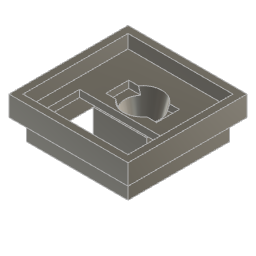
Jet Select Buttons v2 (Autodesk Fusion 360 design; units mm, degrees)
Autodesk Fusion 360 part; units mm, degrees
sketch "Sketch1" plane through (0, 0, 0) normal (0, 1, 0) x (1, 0, 0) in component "PUSH BUTTON SUPPORT v7"
  line L0 (2.815, 2.25) -> (-2.815, 2.25)
  line L1 (-2.815, 2.25) -> (-2.815, -2.25)
  line L2 (-2.815, -2.25) -> (2.815, -2.25)
  line L3 (2.815, -2.25) -> (2.815, 2.25)
  line L4 (2.815, 2.25) -> (-2.815, -2.25) construction
  line L5 (-2.815, 2.25) -> (2.815, -2.25) construction
  line L6 (3.815, 3.25) -> (-3.815, 3.25)
  line L7 (-3.815, 3.25) -> (-3.815, -3.25)
  line L8 (-3.815, -3.25) -> (3.815, -3.25)
  line L9 (3.815, -3.25) -> (3.815, 3.25)
  line L10 (3.815, 3.25) -> (-3.815, -3.25) construction
  line L11 (-3.815, 3.25) -> (3.815, -3.25) construction
  line L12 (1, 1.85) -> (-1, 1.85)
  line L13 (1, 1.85) -> (-1, -1.85) construction
  line L14 (-1, 1.85) -> (1, -1.85) construction
  line L15 (-0.994265, -2.25) -> (1, -2.25)
  line L16 (1, -2.25) -> (1, -1.85)
  line L17 (1, -1.85) -> (-0.994265, -1.85)
  line L18 (-0.994265, -1.85) -> (-0.994265, -2.25)
  line L19 (1, 1.85) -> (1, 2.25)
  line L20 (1, 2.25) -> (-1, 2.25)
  line L21 (-1, 2.25) -> (-1, 1.85)
  line L22 (-2.815, -2.25) -> (-2.515, -2.25)
  line L23 (-2.515, -2.25) -> (-2.515, 2.25)
  line L24 (-2.515, 2.25) -> (-2.815, 2.25)
  line L25 (-2.815, 2.25) -> (-2.815, -2.25)
  line L26 (2.815, -2.25) -> (2.515, -2.25)
  line L27 (2.515, -2.25) -> (2.515, 2.25)
  line L28 (2.515, 2.25) -> (2.815, 2.25)
  line L29 (2.815, 2.25) -> (2.815, -2.25)
  dimension "d1" = 5.63
  dimension "d2" = 4.5
  dimension "d3" = 7.63
  dimension "d4" = 6.5
  dimension "d7" = 2
  dimension "d8" = 3.7
  dimension "d11" = 0.3
  dimension "d12" = 0.3
  constraint horizontal L0
  constraint perpendicular L0 L1
  constraint parallel L0 L2
  constraint parallel L1 L3
  constraint coincident L4 origin
  constraint coincident L5 origin
  constraint horizontal L6
  constraint perpendicular L6 L7
  constraint parallel L6 L8
  constraint parallel L7 L9
  constraint coincident L10 origin
  constraint coincident L11 origin
  constraint horizontal L12
  constraint coincident L13 origin
  constraint coincident L14 origin
  constraint horizontal L15
  constraint vertical L16
  constraint horizontal L17
  constraint vertical L18
  constraint vertical L19
  constraint horizontal L20
  constraint vertical L21
  constraint coincident L0 L19.end
  constraint horizontal L22
  constraint vertical L23
  constraint horizontal L24
  constraint vertical L25
  constraint horizontal L26
  constraint vertical L27
  constraint horizontal L28
  constraint vertical L29
  measures "d1" distance of L1.end L2.end
  measures "d2" distance of L0.end L1.end
  measures "d3" distance of L7.end L8.end
  measures "d4" distance of L6.end L7.end
  measures "d7" distance of L13.end L14.end
  measures "d8" distance of L12.end L13.end
  measures "d11" distance of L1.end L22.end
  measures "d12" distance of L2.end L26.end
extrude "Extrude1" add sketch "Sketch1" along normal blind 5 contours L6 L7 L8 L9 picked at (-0.331422, -2.916667) in component "PUSH BUTTON SUPPORT v7"
extrude "Extrude2" add sketch "Sketch1" along normal blind 5 contours L0 L12 L19 L20 L21 | L2 L15 L16 L17 L18 picked at (-0.333333, 2.116667) picked at (0.335245, -2.116667) in component "PUSH BUTTON SUPPORT v7"
extrude "Extrude3" add sketch "Sketch1" along normal blind 1.8 contours L0 L2 L3 L26 L27 L28 L29 | L0 L1 L2 L22 L23 L24 L25 picked at (2.615, 0.75) picked at (-2.715, 0.75) in component "PUSH BUTTON SUPPORT v7"
chamfer "Chamfer1" distance 0.3 angle 45 2 edges at (-2.515, 1.8, 0) (2.515, 1.8, 0) in component "PUSH BUTTON SUPPORT v7"
chamfer "Chamfer3" distance 0.9 distance2 0.3 1 edges at (-2.515, 0, 0) measured on face at (-2.515, 0.50002, 0.75) in component "PUSH BUTTON SUPPORT v7"
chamfer "Chamfer4" distance 0.3 distance2 1 1 edges at (2.515, 0, 0) measured on face at (3.381667, 0, 0.75) in component "PUSH BUTTON SUPPORT v7"
sketch "Sketch2" plane through (0, 0, 3.25) normal (0, 0, 1) x (-1, 0, 0) in component "PUSH BUTTON SUPPORT v7"
  line L0 (3.815, 0) -> (-3.815, 0)
  line L1 (-3.815, 0) -> (-3.815, -5)
  line L2 (-3.815, -5) -> (3.815, -5)
  line L3 (3.815, -5) -> (3.815, 0)
  line L4 (-2.81825, -1.967525) -> (2.836671, -1.967525)
  line L5 (2.836671, -1.967525) -> (2.836671, -2.718821)
  line L6 (2.836671, -2.718821) -> (-2.81825, -2.718821)
  line L7 (-2.81825, -2.718821) -> (-2.81825, -1.967525)
  constraint horizontal L4
  constraint vertical L5
  constraint horizontal L6
  constraint vertical L7
extrude "Extrude4" add sketch "Sketch2" against normal blind 6.5 contours L4 L5 L6 L7 picked at (-0.933276, -2.217957) in component "PUSH BUTTON SUPPORT v7"
sketch "Sketch3" plane through (0, 1.967525, 0) normal (0, -1, 0) x (1, 0, 0) in component "PUSH BUTTON SUPPORT v7"
  line L0 (-1, -1.85) -> (1, -1.85)
  line L1 (1, -1.85) -> (1, -2.25)
  line L2 (1, -2.25) -> (2.815, -2.25)
  line L3 (2.815, -2.25) -> (2.815, 2.25)
  line L4 (2.815, 2.25) -> (1, 2.25)
  line L5 (1, 2.25) -> (1, 1.85)
  line L6 (1, 1.85) -> (-0.994265, 1.85)
  line L7 (-0.994265, 1.85) -> (-0.994265, 2.25)
  line L8 (-0.994265, 2.25) -> (-2.815, 2.25)
  line L9 (-2.815, 2.25) -> (-2.815, -2.25)
  line L10 (-2.815, -2.25) -> (-1, -2.25)
  line L11 (-1, -2.25) -> (-1, -1.85)
  circle A0 centre (0, 0) radius 1.019835
  constraint coincident A0.centre origin
extrude "Extrude5" cut sketch "Sketch3" against normal blind 6.5 contours A0 picked at (-0.371624, 0.422719) in component "PUSH BUTTON SUPPORT v7"
extrude "Extrude6" cut 1 faces at (-0.331422, 5, 2.916667) along direction (0, -1, 0) blind 2 in component "PUSH BUTTON SUPPORT v7"
extrude "Extrude7" cut 1 faces at (1, 0.655842, -1.983333) along direction (-1, 0, 0) blind 0.3 in component "PUSH BUTTON SUPPORT v7"
extrude "Extrude8" cut 1 faces at (1, 0.655842, 2.116667) along direction (-1, 0, 0) blind 0.3 in component "PUSH BUTTON SUPPORT v7"
extrude "Extrude9" cut 1 faces at (-1, 0.655842, -2.116667) along direction (1, 0, 0) blind 0.3 in component "PUSH BUTTON SUPPORT v7"
extrude "Extrude10" cut 1 faces at (-0.994265, 0.655842, 1.983333) along direction (1, 0, 0) blind 0.3 in component "PUSH BUTTON SUPPORT v7"
extrude "Extrude11" cut 2 faces at (-1.305, 0.955842, -2.25) (1.305, 0.989175, -2.25) along direction (0, 0, -1) blind 0.3 in component "PUSH BUTTON SUPPORT v7"
extrude "Extrude12" cut 2 faces at (-1.301176, 0.955842, 2.25) (1.305, 0.989175, 2.25) along direction (0, 0, 1) blind 0.3 in component "PUSH BUTTON SUPPORT v7"
extrude "Extrude13" cut 1 faces at (-3.481667, 0, -0.85) along direction (0, 1, 0) blind 0.5 in component "PUSH BUTTON SUPPORT v7"
extrude "Extrude14" cut 1 faces at (-2.815, 0.166667, -0.85) along direction (1, 0, 0) blind 8 in component "PUSH BUTTON SUPPORT v7"
extrude "Extrude15" cut 2 faces at (2.81498, 1.8, 0.85) (2.71496, 1.70002, -0.85) along direction (0.70710678, -0.70710678, 0) blind 0.3 in component "PUSH BUTTON SUPPORT v7"
extrude "Extrude16" cut 2 faces at (-2.81498, 1.8, -0.85) (-2.71496, 1.70002, -0.85) along direction (-0.70710678, -0.70710678, 0) blind 0.3 in component "PUSH BUTTON SUPPORT v7"
extrude "Extrude17" cut 1 faces at (2.565, 0.833333, 0.85) along direction (0.95782629, 0.28734789, 0) blind 0.1 in component "PUSH BUTTON SUPPORT v7"
extrude "Extrude18" cut 1 faces at (-2.559444, 0.766667, 0.85) along direction (-0.9486833, 0.31622777, 0) blind 0.1 in component "PUSH BUTTON SUPPORT v7"
extrude "Extrude19" cut 1 faces at (2.515, 1.166687, 0.85) along direction (1, 0, 0) blind 0.1 in component "PUSH BUTTON SUPPORT v7"
extrude "Extrude20" cut 1 faces at (-2.515, 1.10002, 0.85) along direction (-1, 0, 0) blind 0.1 in component "PUSH BUTTON SUPPORT v7"
extrude "Extrude21" cut 1 faces at (-2.815, 1.911683, -0.85) along direction (-1, 0, 0) blind 0.2 in component "PUSH BUTTON SUPPORT v7"
extrude "Extrude22" cut 1 faces at (2.815, 1.911683, -0.85) along direction (1, 0, 0) blind 0.2 in component "PUSH BUTTON SUPPORT v7"
extrude "Extrude23" cut 1 faces at (-0.7, 0.989175, -2.316667) along direction (1, 0, 0) blind 0.5 in component "PUSH BUTTON SUPPORT v7"
extrude "Extrude24" cut 1 faces at (-0.694265, 1.47835, 2.316667) along direction (1, 0, 0) blind 0.5 in component "PUSH BUTTON SUPPORT v7"
extrude "Extrude25" cut 1 faces at (0.7, 0.989175, 2.316667) along direction (-1, 0, 0) blind 0.5 in component "PUSH BUTTON SUPPORT v7"
extrude "Extrude26" cut 1 faces at (0.7, 1.47835, -2.316667) along direction (-1, 0, 0) blind 0.5 in component "PUSH BUTTON SUPPORT v7"
extrude "Extrude27" cut 1 faces at (0.068578, 0.989175, 1.85) along direction (0, 0, 1) blind 0.2 in component "PUSH BUTTON SUPPORT v7"
extrude "Extrude28" cut 1 faces at (0.066667, 0.989175, -1.85) along direction (0, 0, -1) blind 0.2 in component "PUSH BUTTON SUPPORT v7"
extrude "Extrude29" cut 2 faces at (1.005, 1.289195, -2.55) (-1.005, 1.289195, -2.55) along direction (0, 0, -1) blind 0.1 in component "PUSH BUTTON SUPPORT v7"
extrude "Extrude30" cut 2 faces at (-1.001176, 1.289195, 2.55) (1.005, 1.289195, 2.55) along direction (0, 0, 1) blind 0.1 in component "PUSH BUTTON SUPPORT v7"
chamfer "Chamfer2" [suppressed] in component "PUSH BUTTON SUPPORT v7"
sketch "Sketch1 (2)" plane through (0, 0, 0.878877) normal (0, 0, 1) x (-1, 0, 0)
  circle A0 centre (0, -1.839996) radius 1.019835
  line L0 (-1, -3.689996) -> (1, -3.689996)
  line L1 (1, -3.689996) -> (1, -4.089996)
  line L2 (1, -4.089996) -> (2.815, -4.089996)
  line L3 (2.815, -4.089996) -> (2.815, 0.410004)
  line L4 (2.815, 0.410004) -> (0.994265, 0.410004)
  line L5 (0.994265, 0.410004) -> (0.994265, 0.010004)
  line L6 (0.994265, 0.010004) -> (-1, 0.010004)
  line L7 (-1, 0.010004) -> (-1, 0.410004)
  line L8 (-1, 0.410004) -> (-2.815, 0.410004)
  line L9 (-2.815, 0.410004) -> (-2.815, -4.089996)
  line L10 (-2.815, -4.089996) -> (-1, -4.089996)
  line L11 (-1, -4.089996) -> (-1, -3.689996)
  line L12 (2.815, -4.089996) -> (-2.815, -4.089996)
  line L13 (-2.815, -4.089996) -> (-2.815, 0.410004)
  line L14 (-2.815, 0.410004) -> (2.815, 0.410004)
  line L15 (2.815, 0.410004) -> (2.815, -4.089996)
  circle A1 centre (0, -1.839996) radius 1.019835
  constraint horizontal L12
  constraint vertical L13
  constraint horizontal L14
  constraint vertical L15
extrude "Extrude31" add sketch "Sketch1 (2)" along normal blind 0.281 contours L0 L1 L2 L3 L4 L5 L6 L7 L8 L9 L10 L11 L12 L13 L14 L15 picked at (-2.216612, -1.839996) sketch seen with x (1, 0, 0) y (0, 0, -1) z (0, 1, 0) at (0, 1.839944, 1.839996) in component "PUSH BUTTON SUPPORT v7"
sketch "Sketch2 (2)" plane through (0, 0, 1.160056) normal (0, 0, 1) x (-1, 0, 0)
  line L0 (-2.815, -4.089996) -> (-2.815, 0.410004)
  line L1 (-2.815, 0.410004) -> (-1, 0.410004)
  line L2 (-1, 0.410004) -> (-1, 0.010004)
  line L3 (-1, 0.010004) -> (0.994265, 0.010004)
  line L4 (0.994265, 0.010004) -> (0.994265, 0.410004)
  line L5 (0.994265, 0.410004) -> (2.815, 0.410004)
  line L6 (2.815, 0.410004) -> (2.815, -4.089996)
  line L7 (2.815, -4.089996) -> (1, -4.089996)
  line L8 (1, -4.089996) -> (1, -3.689996)
  line L9 (1, -3.689996) -> (-1, -3.689996)
  line L10 (-1, -3.689996) -> (-1, -4.089996)
  line L11 (-1, -4.089996) -> (-2.815, -4.089996)
  line L12 (-3.815, 1.410004) -> (-3.815, -5.089996)
  line L13 (-3.815, -5.089996) -> (3.815, -5.089996)
  line L14 (3.815, -5.089996) -> (3.815, 1.410004)
  line L15 (3.815, 1.410004) -> (-3.815, 1.410004)
  line L16 (0.003684, -1.88932) -> (2.866211, -1.88932)
  line L17 (2.866211, -1.88932) -> (2.866211, -7.811173)
  line L18 (2.866211, -7.811173) -> (0.003684, -7.811173)
  line L19 (0.003684, -7.811173) -> (0.003684, -1.88932)
  line L20 (0.003684, -1.88932) -> (-1.123776, -1.88932)
  line L21 (-1.123776, -1.88932) -> (-1.123776, 8.11068)
  line L22 (-1.123776, 8.11068) -> (0.003684, 8.11068)
  line L23 (0.003684, 8.11068) -> (0.003684, -1.88932)
  line L24 (-4.246316, 1.795447) -> (4.253684, 1.795447)
  line L25 (4.253684, 1.795447) -> (4.253684, -5.574087)
  line L26 (4.253684, -5.574087) -> (-4.246316, -5.574087)
  line L27 (-4.246316, -5.574087) -> (-4.246316, 1.795447)
  line L28 (-4.246316, 1.795447) -> (4.253684, -5.574087) construction
  line L29 (4.253684, 1.795447) -> (-4.246316, -5.574087) construction
  line L30 (8.540865, -7.770507) -> (-8.459135, -7.770507)
  line L31 (-8.459135, -7.770507) -> (-8.459135, 9.229493)
  line L32 (-8.459135, 9.229493) -> (8.540865, 9.229493)
  line L33 (8.540865, 9.229493) -> (8.540865, -7.770507)
  point P0 (0.003684, -1.88932)
  dimension "d78" = 10
  dimension "d79" = 8.5
  dimension "d80" = 17
  dimension "d81" = 17
  constraint horizontal L16
  constraint vertical L17
  constraint horizontal L18
  constraint vertical L19
  constraint horizontal L20
  constraint vertical L21
  constraint horizontal L22
  constraint vertical L23
  constraint horizontal L24
  constraint perpendicular L24 L25
  constraint parallel L24 L26
  constraint parallel L25 L27
  constraint horizontal L30
  constraint vertical L31
  constraint horizontal L32
  constraint vertical L33
extrude "Extrude32" add sketch "Sketch2 (2)" along normal blind 4 contours L0 L1 L9 L10 L11 L12 L13 L15 L19 L21 | L0 L1 L9 L10 L11 L19 L20 L21 | L1 L2 L3 L15 L21 L23 | L1 L2 L3 L20 L21 L23 | L15 L21 L23 L24 | L12 L13 L15 L19 L21 L24 L26 L27 | L6 L7 L8 L9 L16 L19 | L6 L7 L8 L9 L13 L16 L17 L19 | L3 L4 L5 L6 L16 L23 | L13 L14 L15 L17 L23 L24 L25 L26 | L3 L4 L5 L6 L13 L14 L15 L16 L17 L23 | L17 L19 L21 L22 L23 L24 L25 L26 L27 L30 L31 L32 L33 | L21 L22 L23 L24 | L13 L17 L19 L26 | L17 L19 L26 L30 picked at (-3.481667, -1.089996) picked at (-2.251259, -1.856437) picked at (-0.330878, 0.610004) picked at (-0.706697, -1.256212) picked at (-0.372136, 1.538485) picked at (-2.685878, -5.412723) picked at (1.272895, -2.489545) picked at (1.289965, -4.756662) picked at (1.270983, -1.256212) picked at (4.107456, -2.956212) picked at (3.498737, -1.856437) picked at (4.266077, 6.37854) picked at (-0.372136, 6.005602) picked at (0.957859, -5.251359) picked at (1.912035, -7.038367) sketch seen with x (1, 0, 0) y (0, 0, -1) z (0, 1, 0) at (0, 1.839944, 1.839996) in component "PUSH BUTTON SUPPORT v7"
extrude "Extrude33" cut 1 faces at (-1.29891, 3, 8.462992) along direction (0, 1, 0) blind 3 in component "PUSH BUTTON SUPPORT v7"
extrude "Extrude34" cut 1 faces at (2.792469, 6.333333, 11.069488) along direction (0, 0, -1) blind 0.5 in component "PUSH BUTTON SUPPORT v7"
extrude "Extrude35" add 1 faces at (-2.874198, 6.333333, -5.930512) along direction (0, 0, -1) blind 0.5 in component "PUSH BUTTON SUPPORT v7"
sketch "Sketch3 (2)" plane through (0, 0, 5.160056) normal (0, 0, 1) x (-1, 0, 0)
  line L0 (8.540865, 8.729493) -> (-8.459135, 8.729493)
  line L1 (-8.459135, 8.729493) -> (-8.459135, -8.270507)
  line L2 (-8.459135, -8.270507) -> (8.540865, -8.270507)
  line L3 (8.540865, -8.270507) -> (8.540865, 8.729493)
  line L4 (5.982549, 1.207457) -> (-6.017451, 1.207457)
  line L5 (-6.017451, 1.207457) -> (-6.017451, 7.707457)
  line L6 (-6.017451, 7.707457) -> (5.982549, 7.707457)
  line L7 (5.982549, 7.707457) -> (5.982549, 1.207457)
  line L8 (5.982549, 1.207457) -> (-6.017451, 7.707457) construction
  line L9 (-6.017451, 1.207457) -> (5.982549, 7.707457) construction
  point P0 (-0.017451, 4.457457)
  dimension "d90" = 12
  dimension "d91" = 6.5
  constraint horizontal L4
  constraint perpendicular L4 L5
  constraint parallel L4 L6
  constraint parallel L5 L7
extrude "Extrude36" cut sketch "Sketch3 (2)" against normal blind 1 contours L4 L5 L6 L7 picked at (1.982549, 3.374123) sketch seen with x (1, 0, 0) y (0, 0, -1) z (0, 1, 0) at (0, 1.839944, 1.839996) in component "PUSH BUTTON SUPPORT v7"
sketch "Sketch4" plane through (0, 0, 5.160056) normal (0, 0, 1) x (-1, 0, 0)
  line L0 (-6.017451, 1.207457) -> (-6.017451, 7.707457)
  line L1 (-6.017451, 7.707457) -> (5.982549, 7.707457)
  line L2 (5.982549, 7.707457) -> (5.982549, 1.207457)
  line L3 (5.982549, 1.207457) -> (-6.017451, 1.207457)
  line L4 (8.540865, 8.729493) -> (-8.459135, 8.729493)
  line L5 (-8.459135, 8.729493) -> (-8.459135, -8.270507)
  line L6 (-8.459135, -8.270507) -> (8.540865, -8.270507)
  line L7 (8.540865, -8.270507) -> (8.540865, 8.729493)
  circle A0 centre (-0.005434, -1.819158) radius 1.75
  dimension "d94" = 3.5
  measures "d94" diameter of A0
extrude "Extrude37" cut sketch "Sketch4" against normal blind 6 contours A0 picked at (-0.585359, -1.346886) sketch seen with x (1, 0, 0) y (0, 0, -1) z (0, 1, 0) at (0, 1.839944, 1.839996) in component "PUSH BUTTON SUPPORT v7"
sketch "Sketch5" plane through (0, 0, 5.160056) normal (0, 0, 1) x (-1, 0, 0)
  circle A0 centre (-0.005434, -1.819158) radius 1.75
  line L0 (-6.017451, 1.207457) -> (-6.017451, 7.707457)
  line L1 (-6.017451, 7.707457) -> (5.982549, 7.707457)
  line L2 (5.982549, 7.707457) -> (5.982549, 1.207457)
  line L3 (5.982549, 1.207457) -> (-6.017451, 1.207457)
  line L4 (8.540865, 8.729493) -> (-8.459135, 8.729493)
  line L5 (-8.459135, 8.729493) -> (-8.459135, -8.270507)
  line L6 (-8.459135, -8.270507) -> (8.540865, -8.270507)
  line L7 (8.540865, -8.270507) -> (8.540865, 8.729493)
  line L8 (8.540865, -8.270507) -> (-8.459135, -8.270507)
  line L9 (-8.459135, -8.270507) -> (-8.459135, 8.729493)
  line L10 (-8.459135, 8.729493) -> (8.540865, 8.729493)
  line L11 (8.540865, 8.729493) -> (8.540865, -8.270507)
  line L12 (8.540865, -8.270507) -> (-8.459135, 8.729493)
  line L13 (-8.459135, -8.270507) -> (8.540865, 8.729493)
  line L14 (7.540865, -7.270507) -> (-7.459135, -7.270507)
  line L15 (-7.459135, -7.270507) -> (-7.459135, 7.729493)
  line L16 (-7.459135, 7.729493) -> (7.540865, 7.729493)
  line L17 (7.540865, 7.729493) -> (7.540865, -7.270507)
  line L18 (7.540865, -7.270507) -> (-7.459135, 7.729493) construction
  line L19 (-7.459135, -7.270507) -> (7.540865, 7.729493) construction
  point P0 (0.040865, 0.229493)
  dimension "d97" = 15
  dimension "d98" = 15
  constraint horizontal L8
  constraint vertical L9
  constraint horizontal L10
  constraint vertical L11
  constraint horizontal L14
  constraint perpendicular L14 L15
  constraint parallel L14 L16
  constraint parallel L15 L17
extrude "Extrude38" add sketch "Sketch5" along normal blind 1.9 contours L7 L11 L12 L13 L17 | L6 L8 L12 L13 L14 | L5 L9 L12 L13 L15 | L4 L10 L12 L13 L16 picked at (8.207531, -2.270507) picked at (-2.459135, -7.937174) picked at (-8.125802, 2.729493) picked at (-2.459135, 8.396159) sketch seen with x (1, 0, 0) y (0, 0, -1) z (0, 1, 0) at (0, 1.839944, 1.839996) in component "PUSH BUTTON SUPPORT v7"
extrude "Extrude39" add 1 faces at (2.017451, 6.666667, 9.547452) along direction (0, 0, -1) blind 1 in component "PUSH BUTTON SUPPORT v7"
chamfer "Chamfer5" distance 1 distance2 4 1 edges at (1.637007, 7, 0.653665) measured on face at (-5.082811, 7, -0.874348) in component "PUSH BUTTON SUPPORT v7"
sketch "Sketch6" plane through (0, 0, 5.160056) normal (0, 0, 1) x (-1, 0, 0)
  line L0 (-6.017451, 1.207457) -> (-6.017451, 6.707457)
  line L1 (-6.017451, 6.707457) -> (5.982549, 6.707457)
  line L2 (5.982549, 6.707457) -> (5.982549, 1.207457)
  line L3 (5.982549, 1.207457) -> (-6.017451, 1.207457)
  line L4 (-7.459135, 7.729493) -> (-7.459135, -7.270507)
  line L5 (-7.459135, -7.270507) -> (7.540865, -7.270507)
  line L6 (7.540865, -7.270507) -> (7.540865, 7.729493)
  line L7 (7.540865, 7.729493) -> (-7.459135, 7.729493)
  circle A0 centre (-0.005434, -1.819158) radius 2.75
  line L8 (3.614753, -3.441837) -> (-3.625622, -3.441837)
  line L9 (-3.625622, -3.441837) -> (-3.625622, -0.196479)
  line L10 (-3.625622, -0.196479) -> (3.614753, -0.196479)
  line L11 (3.614753, -0.196479) -> (3.614753, -3.441837)
  line L12 (3.614753, -3.441837) -> (-3.625622, -0.196479) construction
  line L13 (-3.625622, -3.441837) -> (3.614753, -0.196479) construction
  point P0 (-0.005434, -1.819158)
  constraint horizontal L8
  constraint perpendicular L8 L9
  constraint parallel L8 L10
  constraint parallel L9 L11
extrude "Extrude40" cut sketch "Sketch6" against normal blind 1 contours A0 L8 L10 | A0 L8 L10 L11 | A0 L8 L9 L10 picked at (-0.80412, -1.149714) picked at (3.32469, -1.819158) picked at (-3.333306, -1.754928) sketch seen with x (1, 0, 0) y (0, 0, -1) z (0, 1, 0) at (0, 1.839944, 1.839996) in component "PUSH BUTTON SUPPORT v7"
sketch "Sketch7" plane through (0, 0, 4.160056) normal (0, 0, -1) x (1, 0, 0)
  line L0 (6.017451, 1.207457) -> (3.815, 1.207457)
  line L1 (3.815, 1.207457) -> (3.815, -5.089996)
  line L2 (3.815, -5.089996) -> (-3.815, -5.089996)
  line L3 (-3.815, -5.089996) -> (-3.815, 1.207457)
  line L4 (-3.815, 1.207457) -> (-5.982549, 1.207457)
  line L5 (-5.982549, 1.207457) -> (-5.982549, 6.707457)
  line L6 (-5.982549, 6.707457) -> (6.017451, 6.707457)
  line L7 (6.017451, 6.707457) -> (6.017451, 1.207457)
  line L8 (8.459135, 8.729493) -> (-8.540865, 8.729493)
  line L9 (-8.540865, 8.729493) -> (-8.540865, -8.270507)
  line L10 (-8.540865, -8.270507) -> (8.459135, -8.270507)
  line L11 (8.459135, -8.270507) -> (8.459135, 8.729493)
  line L12 (-8.540865, 8.729493) -> (8.459135, -8.270507)
  line L13 (8.459135, 8.729493) -> (-8.540865, -8.270507)
  line L14 (-7.290865, 7.479493) -> (7.209135, 7.479493)
  line L15 (7.209135, 7.479493) -> (7.209135, -7.020507)
  line L16 (7.209135, -7.020507) -> (-7.290865, -7.020507)
  line L17 (-7.290865, -7.020507) -> (-7.290865, 7.479493)
  line L18 (-7.290865, 7.479493) -> (7.209135, -7.020507) construction
  line L19 (7.209135, 7.479493) -> (-7.290865, -7.020507) construction
  line L20 (6.709135, 6.979493) -> (-6.790865, 6.979493)
  line L21 (-6.790865, 6.979493) -> (-6.790865, -6.520507)
  line L22 (-6.790865, -6.520507) -> (6.709135, -6.520507)
  line L23 (6.709135, -6.520507) -> (6.709135, 6.979493)
  line L24 (6.709135, 6.979493) -> (-6.790865, -6.520507) construction
  line L25 (-6.790865, 6.979493) -> (6.709135, -6.520507) construction
  point P0 (-0.040865, 0.229493)
  point P1 (-0.040865, 0.229493)
  dimension "d107" = 14.5
  dimension "d108" = 14.5
  dimension "d109" = 13.5
  dimension "d110" = 13.5
  constraint horizontal L14
  constraint perpendicular L14 L15
  constraint parallel L14 L16
  constraint parallel L15 L17
  constraint horizontal L20
  constraint perpendicular L20 L21
  constraint parallel L20 L22
  constraint parallel L21 L23
extrude "Extrude41" add sketch "Sketch7" along normal blind 3 contours L12 L13 L14 L20 | L12 L13 L15 L23 | L12 L13 L16 L22 | L12 L13 L17 L21 picked at (2.209135, 7.312826) picked at (7.042469, 2.479493) picked at (2.209135, -6.853841) picked at (-7.124198, -2.020507) sketch seen with x (1, 0, 0) y (0, 0, -1) z (0, 1, 0) at (0, 1.839944, 1.839996) in component "PUSH BUTTON SUPPORT v7"
component "PUSH BUTTON SUPPORT v7" placed x (1, 0, 0) y (0, 0, 1) z (0, -1, 0) at (0, 1.839996, -1.839944)
